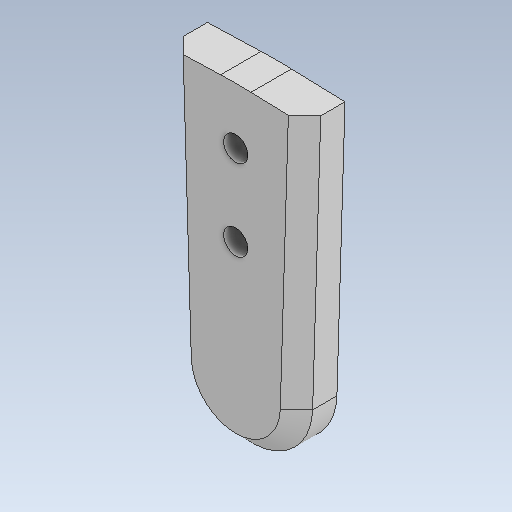
# Autodesk Inventor part: leg_bone_2
Saved by Autodesk Inventor 2020 (Build 240168000, 168)
## iProperties
Created: 2019-04-28
Part Number: leg_bone_2
Material: Generic
Document SubType Name: Modeling
Designer: psrob
Density: 1 g/cm^3
Appearance: Default
Author: psrob
Autodesk Inventor part; units mm, degrees
ref_plane "YZ Plane" through (0, 0, 0) normal (1, 0, 0) x (0, 1, 0)
ref_plane "XZ Plane" through (0, 0, 0) normal (0, 1, 0) x (-1, 0, 0)
ref_plane "XY Plane" through (0, 0, 0) normal (0, 0, 1) x (1, 0, 0)
sketch "Sketch1" plane through (0, 0, 0) normal (0, 0, 1) x (1, 0, 0)
  line L0 (-4.4434, -31.1874) -> (-7.8728, -29.4435) projected
  arc A0 (4.4434, -31.1874) -> (-4.4434, -31.1874) centre (0, -41.25) ccw projected
  line L1 (7.8728, -29.4435) -> (4.4434, -31.1874) projected
  line L2 (7.8728, -29.4435) -> (9.9951, 38.4375) projected
  arc A1 (9.9951, 38.4375) -> (-9.9951, 38.4375) centre (0, 38.75) ccw projected
  line L3 (-9.9951, 38.4375) -> (-7.8728, -29.4435) projected
  circle A2 centre (0, -26.25) radius 1.5 projected
  circle A3 centre (0, -16.25) radius 1.5 projected
  circle A4 centre (0, -41.25) radius 7.5
  line L4 (0, -16.25) -> (0, -9.25)
  line L5 (0, -9.25) -> (8.4958, -9.5156)
  line L6 (0, -9.25) -> (-8.4958, -9.5156)
  line L7 (0, -41.25) -> (7.4963, -41.4844)
  line L8 (0, -41.25) -> (-7.4963, -41.4844)
  line L9 (-8.4958, -9.5156) -> (-7.4963, -41.4844)
  line L10 (7.4963, -41.4844) -> (8.4958, -9.5156)
  arc A5 (-7.4963, -41.4844) -> (7.4963, -41.4844) centre (0, -41.25) ccw
  point P0 (0, 0)
  dimension "d0" = 15
  dimension "d1" = 7
  dimension "d2" = 7.5
  constraints: 14 end point, 4 perpendicular, 2 point on circle, 2 point on line, 1 centre point, 1 coincident, 1 collinear, 1 vertical, 3 other
  measures "d1" distance of L4.start L4.end
  measures "d2" radius of A5
extrude "Extrusion1" add sketch "Sketch1" along normal blind 5 contours A0 L1 L10 A4 L9 L0 | L0 L3 L6 L5 L2 L1 A0 | L8 L7 A4 | A4 L7 L8
chamfer "Chamfer1" distance 2 angle 45 3 edges at (-8.1843, -19.4796, 5) (0, -48.75, 5) (8.1843, -19.4796, 5)
fillet "Fillet1" radius 60 1 edges at (0, -9.25, 2.5)
body "Solid1"
